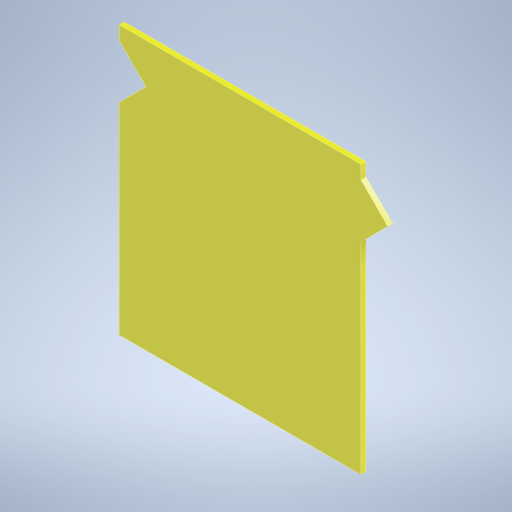
# Autodesk Inventor part: MS_RI_back_v3
Saved by Autodesk Inventor 2024 (Build 280153000, 153)
## iProperties
Created: 2024-02-15
Part Number: MS_RI_back_v3
Material: Generic
Document SubType Name: Modeling
Designer: LKLM
Density: 1 g/cm^3
Appearance: Yellow
Author: LKLM
Autodesk Inventor part; units mm, degrees
ref_plane "YZ Plane" through (0, 0, 0) normal (1, 0, 0) x (0, 1, 0)
ref_plane "XZ Plane" through (0, 0, 0) normal (0, 1, 0) x (-1, 0, 0)
ref_plane "XY Plane" through (0, 0, 0) normal (0, 0, 1) x (1, 0, 0)
sketch "Sketch1" plane through (0, 0, 0) normal (0, 0, 1) x (1, 0, 0)
  line L0 (0, 0) -> (-72, 0)
  circle A0 centre (-72, 68) radius 8 construction
  line L1 (-72, 60) -> (0, 60) construction
  line L2 (-72, 76) -> (-64, 68)
  line L3 (-72, 60) -> (-64, 68)
  line L4 (0, 60) -> (0, 0)
  line L5 (-72, 0) -> (-72, 60)
  line L6 (-72, 76) -> (-72, 80)
  line L7 (0, 76) -> (0, 80)
  line L8 (-72, 80) -> (0, 80)
  line L9 (-72, 76) -> (11.0791, 76) construction
  line L10 (-64, 68) -> (11.3495, 68) construction
  line L11 (-72, 60) -> (22.6598, 60) construction
  circle A1 centre (0, 68) radius 8 construction
  line L12 (0, 60) -> (8, 68)
  line L13 (8, 68) -> (0, 76)
  point P0 (0, 0)
  point P1 (0, 78)
  point P2 (-72, 78)
  dimension "d0" = 80
  dimension "d2" = 60
  dimension "d3" = 0
  dimension "d4" = 0
  dimension "d5" = 72
  constraints: 28 end point, 5 point on circle, 4 horizontal, 4 point on line, 3 parallel, 3 perpendicular, 3 tangent, 2 centre point, 2 midpoint, 1 collinear
  measures "d0" distance of L0.end L8.start
  measures "d2" distance between parallel lines of L0 L1
  measures "d3" distance from line of L0 point (0, 0)
  measures "d4" distance from line of L4 point (0, 0)
  measures "d5" distance of point (0, 78) point (-72, 78)
extrude "Extrusion1" add sketch "Sketch1" along normal blind 1.5
body "Solid1"
